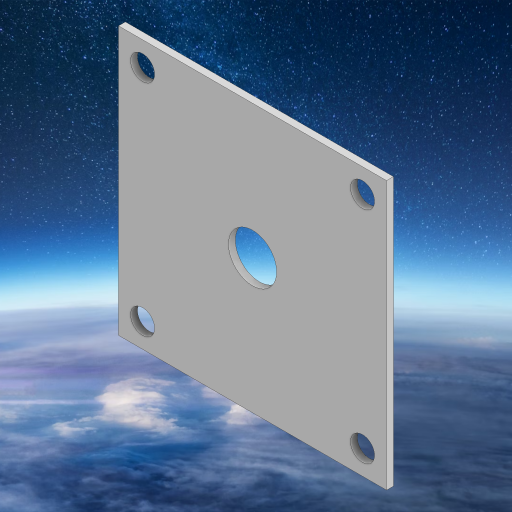
# Autodesk Inventor part: coolingtube_plate
Saved by Autodesk Inventor 2023 (Build 270158000, 158)
## iProperties
Created: 2023-11-17
Part Number: coolingtube_plate
Material: Generic
Document SubType Name: Sheet Metal
Designer: 310611102
Density: 1 g/cm^3
Sheet Metal Rule: Default_mm
Appearance: Default
Author: 310611102
Autodesk Inventor part; units mm, degrees
ref_plane "YZ Plane" through (0, 0, 0) normal (1, 0, 0) x (0, 1, 0)
ref_plane "XZ Plane" through (0, 0, 0) normal (0, 1, 0) x (-1, 0, 0)
ref_plane "XY Plane" through (0, 0, 0) normal (0, 0, 1) x (1, 0, 0)
sketch "Sketch1" plane through (0, 0, 0) normal (0, 0, 1) x (1, 0, 0)
  line L0 (-19.5, 19.5) -> (19.5, 19.5)
  line L1 (19.5, 19.5) -> (19.5, -19.5)
  line L2 (19.5, -19.5) -> (-19.5, -19.5)
  line L3 (-19.5, -19.5) -> (-19.5, 19.5)
  line L4 (-19.5, 19.5) -> (19.5, -19.5) construction
  line L5 (19.5, 19.5) -> (-19.5, -19.5) construction
  circle A0 centre (-16, 16) radius 1.75
  line L6 (0, 0) -> (0, 12.7149)
  line L7 (0, 0) -> (7.8858, 0)
  circle A1 centre (16, 16) radius 1.75
  circle A2 centre (-16, -16) radius 1.75
  circle A3 centre (16, -16) radius 1.75
  circle A4 centre (0, 0) radius 3.5
  dimension "d0" = 39
  dimension "d1" = 39
  dimension "d2" = 3.5
  dimension "d3" = 32
  dimension "d4" = 32
  dimension "d6" = 7
  measures "d0" distance of L0.end L1.end
  measures "d1" distance of L0.start L0.end
  measures "d2" diameter of A0
  measures "d3" distance of A1.centre A0.centre
  measures "d4" distance of A2.centre A0.centre
  measures "d6" diameter of A4
extrude "Plate1" add sketch "Sketch1" along normal blind 1
equation "\"d0\" = d1"
equation "\"d4\" = d3"
equation "\"d5\" = 厚度"
equation "\"折彎半徑\" = 厚度"
equation "\"折彎離隙寬度\" = 厚度"
equation "\"折彎離隙深度\" = 0.5 * 厚度"
equation "\"轉角離隙大小\" = 4 * 厚度"
equation "\"最小剩餘\" = 2 * 厚度"
equation "\"轉移半徑\" = 折彎半徑"
equation "\"Jacobi半徑大小\" = 折彎半徑"
equation "\"間隙大小\" = 厚度"
equation "\"厚度\" = 1"
body "Solid1"
